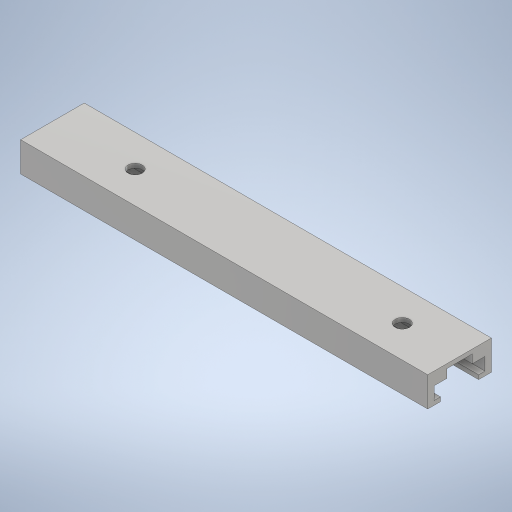
# Autodesk Inventor part: slider2a2
Saved by Autodesk Inventor 2024.1 (Build 281209000, 209)
## iProperties
Created: 2017-08-05
Part Number: slider2a2
Material: アルミニウム 6061-AHC
Document SubType Name: Modeling
Designer: SHUICHI
Density: 2.7 g/cm^3
Appearance: アルミニウム - ダーク
Mass: 11.615 g
Surface Area: 56.6105 cm^2
Volume: 4.30184 cm^3
Author: SHUICHI
Autodesk Inventor part; units mm, degrees
ref_plane "YZ Plane" through (0, 0, 0) normal (1, 0, 0) x (0, 1, 0)
ref_plane "XZ Plane" through (0, 0, 0) normal (0, 1, 0) x (-1, 0, 0)
ref_plane "XY Plane" through (0, 0, 0) normal (0, 0, 1) x (1, 0, 0)
sketch "スケッチ1" plane through (0, 0, 0) normal (1, 0, 0) x (0, 1, 0)
  line L0 (0, 0) -> (15, 0)
  line L1 (15, 0) -> (15, -7)
  line L2 (0, -7) -> (0, 0)
  line L3 (7.5, 0) -> (7.5, -7)
  line L4 (7.5, -1) -> (10.5, -1)
  line L5 (10.5, -1) -> (10.5, -3)
  line L6 (10.5, -3) -> (13.5, -3)
  line L7 (13.5, -3) -> (13.5, -6)
  line L8 (13.5, -6) -> (12, -6)
  line L9 (12, -6) -> (12, -7)
  line L10 (7.5, -1) -> (4.5, -1)
  line L11 (4.5, -1) -> (4.5, -3)
  line L12 (4.5, -3) -> (1.5, -3)
  line L13 (1.5, -3) -> (1.5, -6)
  line L14 (1.5, -6) -> (3, -6)
  line L15 (3, -6) -> (3, -7)
  line L16 (15, -7) -> (12, -7)
  line L17 (3, -7) -> (0, -7)
  dimension "d0" = 15
  dimension "d1" = 7
  dimension "d2" = 3
  dimension "d3" = 2
  dimension "d5" = 3
  dimension "d6" = 3
  dimension "d7" = 1.5
  dimension "d9" = 1
  constraints: 36 end point, 8 perpendicular, 6 symmetric about line, 3 parallel, 1 horizontal, 1 midpoint, 1 point on line
  measures "d0" distance of L1.end L2.start
  measures "d1" distance of L0.end L1.end
  measures "d2" distance of L4.start L4.end
  measures "d3" distance of L4.end L5.end
  measures "d5" distance of L6.end L7.end
  measures "d6" distance between parallel lines of L9 L1
  measures "d7" distance between parallel lines of L1 L7
  measures "d9" distance between parallel lines of L16 L8
extrude "押し出し1" add sketch "スケッチ1" along normal blind 96
sketch "スケッチ2" plane through (0, 0, 0) normal (0, 0, 1) x (1, 0, 0)
  line L0 (0, 4.5) -> (0, 10.5) projected
  line L1 (0, 7.5) -> (96, 7.5)
  line L2 (96, 4.5) -> (96, 10.5) projected
  line L3 (0, 15) -> (0, 0) projected
  line L4 (96, 15) -> (96, 0) projected
  point P0 (19.5, 7.5)
  point P1 (82.5, 7.5)
  dimension "d12" = 19.5
  dimension "d24" = 63
  constraints: 2 end point, 2 midpoint, 2 point on line
  measures "d12" distance from line of L3 point (19.5, 7.5)
  measures "d24" distance of point (82.5, 7.5) point (19.5, 7.5)
hole "穴1" at (19.5, 7.5, 0) at (82.5, 7.5, 0) direction (0, 0, -1) diameter 3.4 end through all
